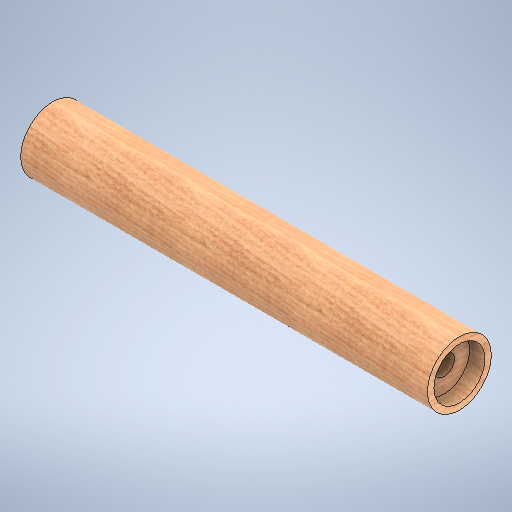
# Autodesk Inventor part: Dowel1
Saved by Autodesk Inventor 2025.3 (Build 293356000, 356)
## iProperties
Created: 2026-01-15
Part Number: Dowel1
Material: Generic
Document SubType Name: Modeling
Designer: Balint
Density: 1 g/cm^3
Appearance: Default
Mass: 66.7977 g
Surface Area: 180.687 cm^2
Volume: 66.7977 cm^3
Author: Balint
Autodesk Inventor part; units mm, degrees
ref_plane "YZ Plane" through (0, 0, 0) normal (1, 0, 0) x (0, 1, 0)
sketch "Sketch1" plane through (0, 0, 0) normal (1, 0, 0) x (0, 1, 0)
  circle A0 centre (0, 0) radius 12.5
  dimension "d0" = 25
  constraints: 1 centre point, 1 coincident
  measures "d0" diameter of A0
extrude "Extrusion1" add sketch "Sketch1" along normal blind 200
ref_plane "Work Plane1" through (0, -12.5, 0) normal (0, 1, 0) x (-1, 0, 0)
sketch "Sketch2" plane through (0, -12.5, 0) normal (0, 1, 0) x (-1, 0, 0)
  line L0 (-200, 12.5) -> (-200, -12.5) projected
  line L1 (-200, 0) -> (-140, 0)
  circle A0 centre (-140, 0) radius 7.5
  point P0 (0, 0)
  dimension "d19" = 60
  dimension "d20" = 15
  constraints: 2 end point, 1 centre point, 1 coincident, 1 horizontal, 1 midpoint
  measures "d19" distance of L1.start L1.end
  measures "d20" diameter of A0
extrude "Extrusion2" cut sketch "Sketch2" along normal blind 15
sketch "Sketch3" plane through (0, 0, 0) normal (-1, 0, 0) x (0, 0, 1)
  line L0 (0, 0) -> (0, -7)
  circle A0 centre (0, -7) radius 2.5
  dimension "d9" = 7
  dimension "d10" = 5
  constraints: 2 end point, 1 centre point, 1 coincident, 1 vertical
  measures "d9" distance of L0.start L0.end
  measures "d10" diameter of A0
extrude "Extrusion3" cut sketch "Sketch3" against normal blind 136
sketch "Sketch4" plane through (200, 0, 0) normal (1, 0, 0) x (0, 0, -1)
  circle A0 centre (0, 0) radius 10
  dimension "d13" = 20
  constraints: 1 centre point, 1 coincident
  measures "d13" diameter of A0
extrude "Extrusion4" cut sketch "Sketch4" against normal blind 6
sketch "Sketch5" plane through (194, 0, 0) normal (1, 0, 0) x (0, 0, -1)
  circle A0 centre (0, 0) radius 4
  dimension "d16" = 8
  constraints: 1 centre point, 1 coincident
  measures "d16" diameter of A0
extrude "Extrusion5" cut sketch "Sketch5" against normal blind 50
sketch "Sketch6" plane through (0, 0, 0) normal (-1, 0, 0) x (0, 0, 1)
  circle A0 centre (0, 0) radius 5
  dimension "d21" = 10
  constraints: 1 centre point, 1 coincident
  measures "d21" diameter of A0
extrude "Extrusion6" cut sketch "Sketch6" against normal blind 80
fillet "Fillet1" radius 0.4 2 edges at (40, -4.8393, 1.2575) (40, -4.8393, -1.2575)
sketch "Sketch7" plane through (0, 0, 0) normal (-1, 0, 0) x (0, 0, 1)
  circle A0 centre (0, 0) radius 38.5321
  constraints: 1 centre point, 1 coincident
extrude "Extrusion7" cut sketch "Sketch7" against normal blind 40
chamfer "Chamfer1" distance 0.4 angle 45 5 edges at (40, 5, 0) (40, -4.9016, 1.691) (40, -4.9016, -1.691) (40, -6.0616, 2.3172) (40, -9.3172, -0.9384)
ref_plane "Work Plane2" through (0, -12.5, 0) normal (0, 1, 0) x (-1, 0, 0)
sketch "Sketch8" plane through (0, -12.5, 0) normal (0, 1, 0) x (-1, 0, 0)
  circle A0 centre (-152.5, 0) radius 1.5
  line L0 (-200, 12.5) -> (-200, -12.5) projected
  point P0 (0, 0)
  dimension "d31" = 3
  dimension "d32" = 47.5
  constraints: 1 centre point
  measures "d31" diameter of A0
  measures "d32" distance from line of A0.centre L0
extrude "Extrusion8" cut sketch "Sketch8" along normal blind 10
body "Solid1"
